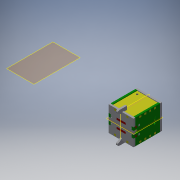
# Autodesk Inventor part: box
Saved by Autodesk Inventor 2019 (Build 230136000, 136)
## iProperties
Created: 2018-09-20
Part Number: box
Material: Générique
Document SubType Name: Modeling
Designer: Jérémy
Density: 1 g/cm^3
Appearance: Par défaut
Author: Jérémy
Autodesk Inventor part; units mm, degrees
(part 1 of 2)
ref_plane "YZ Plane" through (0, 0, 0) normal (1, 0, 0) x (0, 1, 0)
ref_plane "XZ Plane" through (0, 0, 0) normal (0, 1, 0) x (-1, 0, 0)
ref_plane "XY Plane" through (0, 0, 0) normal (0, 0, 1) x (1, 0, 0)
sketch "Esquisse1" plane through (0, 0, 0) normal (0, 0, 1) x (1, 0, 0)
  line L0 (0, 11.8) -> (0, 9.4) projected
  line L1 (0, 11.8) -> (-8.8, 11.8) construction
  line L2 (-8.8, 0) -> (-8.8, 11.8) construction
  line L3 (0, 0) -> (-8.8, 0) projected
  line L4 (0, 2.4) -> (0, 0) projected
  line L5 (0, 2.4) -> (19.5, 2.4) projected
  line L6 (19.5, 9.4) -> (19.5, 2.4) projected
  line L7 (0, 9.4) -> (19.5, 9.4) projected
  line L8 (64, 0) -> (64, 2.4) projected
  line L9 (64, 0) -> (72.8, 0) projected
  line L10 (72.8, 11.8) -> (72.8, 0) construction
  line L11 (64, 11.8) -> (72.8, 11.8) construction
  line L12 (64, 9.4) -> (64, 11.8) projected
  line L13 (64, 9.4) -> (44.5, 9.4) projected
  line L14 (44.5, 2.4) -> (44.5, 9.4) projected
  line L15 (64, 2.4) -> (44.5, 2.4) projected
  line L16 (19.5, 9.4) -> (19.5, 5.9) construction
  line L17 (19.5, 5.9) -> (19.5, 2.4) construction
  line L18 (19.5, 9.4) -> (32, 9.4) construction
  line L19 (32, 9.4) -> (44.5, 9.4) construction
  line L20 (-27.9434, 5.9) -> (85.3545, 5.9) construction
  line L21 (32, 17.9523) -> (32, -8.6548) construction
  line L22 (-8.8, 5.9) -> (-8.8, 11.8)
  line L23 (-2.8, 11.8) -> (-2.8, 21.9)
  line L24 (-2.8, 21.9) -> (17, 21.9)
  line L25 (17, 21.9) -> (17, 15.9)
  line L26 (17, 15.9) -> (32, 15.9)
  line L27 (-2.8, 11.8) -> (-8.8, 11.8)
  circle A0 centre (0.2, 14.8) radius 1.5
  line L28 (64, 11.8) -> (72.8, 11.8) construction
  line L29 (72.8, 0) -> (72.8, 11.8) construction
  line L30 (72.8, 5.9) -> (72.8, 11.8)
  line L31 (66.8, 11.8) -> (66.8, 21.9)
  line L32 (66.8, 21.9) -> (47, 21.9)
  line L33 (47, 21.9) -> (47, 15.9)
  line L34 (47, 15.9) -> (32, 15.9)
  line L35 (66.8, 11.8) -> (72.8, 11.8)
  circle A1 centre (63.8, 14.8) radius 1.5
  line L36 (0, 0) -> (-8.8, 0) construction
  line L37 (64, 0) -> (72.8, 0) construction
  line L38 (-8.8, 5.9) -> (-8.8, 0)
  line L39 (-2.8, 0) -> (-2.8, -10.1)
  line L40 (-2.8, -10.1) -> (17, -10.1)
  line L41 (17, -10.1) -> (17, -4.1)
  line L42 (17, -4.1) -> (32, -4.1)
  line L43 (-2.8, 0) -> (-8.8, 0)
  circle A2 centre (0.2, -3) radius 1.5
  line L44 (64, 0) -> (72.8, 0) construction
  line L45 (66.8, -10.1) -> (47, -10.1)
  line L46 (47, -4.1) -> (32, -4.1)
  line L47 (47, -10.1) -> (47, -4.1)
  circle A3 centre (63.8, -3) radius 1.5
  line L48 (66.8, 0) -> (66.8, -10.1)
  line L49 (66.8, 0) -> (72.8, 0)
  line L50 (72.8, 5.9) -> (72.8, 0)
  point P0 (19.5, 5.9)
  dimension "d0" = 6
  dimension "d1" = 15
  dimension "d2" = 6
  dimension "d3" = 16
  dimension "d4" = 3
  dimension "d5" = 3
  dimension "d6" = 3
  constraints: 70 end point, 17 symmetric about line, 8 point on line, 6 collinear, 4 centre point, 4 perpendicular, 3 midpoint, 2 coincident, 1 horizontal, 1 parallel, 1 vertical, 3 other
  measures "d0" distance of L1.end L23.start
  measures "d1" distance of L25.end L26.end
  measures "d2" distance of L24.end L25.end
  measures "d3" vertical distance of L22.start L23.end
  measures "d4" diameter of A0
  measures "d5" vertical distance of L0.start A0.centre
  measures "d6" horizontal distance of L23.start A0.centre
extrude "Extrusion1" add sketch "Esquisse1" along normal blind 6
ref_plane "Plan de construction1" through (5, 11.8, -9.8) normal (0, 0, -1) x (-1, 0, 0)
sketch "Esquisse2" plane through (5, 11.8, -9.8) normal (0, 0, -1) x (-1, 0, 0)
  circle A0 centre (-58.8, -14.8) radius 1.5 projected
  circle A1 centre (4.8, -14.8) radius 1.5 projected
  circle A2 centre (-58.8, 3) radius 1.5 projected
  circle A3 centre (4.8, 3) radius 1.5 projected
  line L0 (13.8, 0) -> (13.8, -11.8) construction
  line L1 (7.8, 0) -> (13.8, 0) construction
  line L2 (7.8, 10.1) -> (7.8, 0) projected
  line L3 (-12, 10.1) -> (7.8, 10.1) projected
  line L4 (-12, 4.1) -> (-12, 10.1) projected
  line L5 (-42, 4.1) -> (-12, 4.1) projected
  line L6 (-42, 10.1) -> (-42, 4.1) projected
  line L7 (-61.8, 10.1) -> (-42, 10.1) projected
  line L8 (-61.8, 0) -> (-61.8, 10.1) construction
  line L9 (-67.8, 0) -> (-61.8, 0) construction
  line L10 (-67.8, -11.8) -> (-67.8, 0) projected
  line L11 (-61.8, -11.8) -> (-67.8, -11.8) construction
  line L12 (-61.8, -21.9) -> (-61.8, -11.8) construction
  line L13 (-42, -21.9) -> (-61.8, -21.9) projected
  line L14 (-42, -15.9) -> (-42, -21.9) projected
  line L15 (-12, -15.9) -> (-42, -15.9) construction
  line L16 (-12, -21.9) -> (-12, -15.9) projected
  line L17 (7.8, -21.9) -> (-12, -21.9) projected
  line L18 (7.8, -11.8) -> (7.8, -21.9) construction
  line L19 (13.8, -11.8) -> (7.8, -11.8) construction
  line L20 (-67.8, -11.8) -> (-67.8, 0) construction
  line L21 (-67.8, -11.8) -> (-67.8, -5.9) construction
  line L22 (-67.8, -5.9) -> (-67.8, 0) construction
  line L23 (23.1291, -5.9) -> (-93.9049, -5.9) construction
  line L24 (-12, -15.9) -> (-42, -15.9) construction
  line L25 (-12, -15.9) -> (-27, -15.9) construction
  line L26 (-27, -15.9) -> (-42, -15.9) construction
  line L27 (-27, -48.0449) -> (-27, 22.4449) construction
  line L28 (13.8, -21.4) -> (13.8, -16.4)
  line L29 (7.8, -21.9) -> (-12, -21.9) projected
  line L30 (13.3, -21.9) -> (-12, -21.9)
  line L31 (-12, -21.9) -> (-12, -15.9)
  line L32 (-27, -15.9) -> (-12, -15.9)
  line L33 (-12, -15.9) -> (18.1212, -15.9) construction
  line L34 (-9.5, -11.8) -> (-9.5, 0) construction
  line L35 (-9.5, 0) -> (-14.5, 0) construction
  line L36 (-14.5, -11.8) -> (-14.5, 0) construction
  line L37 (-9.5, -11.8) -> (-14.5, -11.8) construction
  line L38 (-44.5, 0) -> (-44.5, -11.8) construction
  line L39 (-44.5, -11.8) -> (-39.5, -11.8) construction
  line L40 (-39.5, 0) -> (-39.5, -11.8) construction
  line L41 (-44.5, 0) -> (-39.5, 0) construction
  line L42 (-27, -12.8) -> (-7.5, -12.8)
  line L43 (-7.5, -12.8) -> (-7.5, -12.8)
  line L44 (-7.5, -12.8) -> (-7.5, -5.9)
  circle A4 centre (-58.8, -14.8) radius 1.5
  line L45 (-42, -15.9) -> (-12, -15.9) construction
  line L46 (-42, -21.9) -> (-42, -15.9)
  line L47 (-61.8, -21.9) -> (-42, -21.9)
  line L48 (-42, -15.9) -> (-12, -15.9) construction
  line L49 (-42, -15.9) -> (-27, -15.9) construction
  line L50 (-67.3, -21.9) -> (-42, -21.9)
  line L51 (-27, -15.9) -> (-42, -15.9)
  line L52 (-27, -12.8) -> (-46.5, -12.8)
  line L53 (-46.5, -12.8) -> (-46.5, -5.9)
  circle A5 centre (-58.8, 3) radius 1.5
  circle A6 centre (4.8, 3) radius 1.5
  line L54 (-42.5, 10.1) -> (-61.8, 10.1)
  line L55 (-42, 4.1) -> (-42, 9.6)
  line L56 (-12, 9.6) -> (-12, 4.1)
  line L57 (7.8, 10.1) -> (-11.5, 10.1)
  line L58 (7.8, 0) -> (7.8, 10.1) construction
  line L59 (-12, 4.1) -> (-27, 4.1) construction
  line L60 (7.8, 10.1) -> (-12, 10.1)
  line L61 (13.3, 10.1) -> (-12, 10.1)
  line L62 (-12, 10.1) -> (-12, 4.1)
  line L63 (-27, 4.1) -> (-12, 4.1)
  line L64 (-27, 1) -> (-7.5, 1)
  line L65 (-7.5, 1) -> (-7.5, -5.9)
  line L66 (-27, 4.1) -> (-42, 4.1)
  line L67 (-67.3, 10.1) -> (-42, 10.1)
  line L68 (-46.5, 1) -> (-46.5, -5.9)
  line L69 (-27, 1) -> (-46.5, 1)
  circle A7 centre (-58.8, 3) radius 1.5
  line L70 (7.8, -5.9) -> (7.8, -15.9)
  line L71 (7.8, -11.8) -> (7.8, -21.9) construction
  line L72 (13.3, -15.9) -> (7.8, -15.9)
  line L73 (-67.8, -21.4) -> (-67.8, -16.4)
  line L74 (-61.8, -5.9) -> (-61.8, -15.9)
  line L75 (-67.3, -15.9) -> (-61.8, -15.9)
  line L76 (13.8, 9.6) -> (13.8, 4.6)
  line L77 (7.8, -5.9) -> (7.8, 4.1)
  line L78 (13.3, 4.1) -> (7.8, 4.1)
  line L79 (-67.8, 9.6) -> (-67.8, 4.6)
  line L80 (-67.3, 4.1) -> (-61.8, 4.1)
  line L81 (-61.8, -5.9) -> (-61.8, 4.1)
  line L82 (-67.3, -21.9) -> (-67.8, -21.4)
  line L83 (-67.8, -16.4) -> (-67.3, -15.9)
  line L84 (-67.3, 4.1) -> (-67.8, 4.6)
  line L85 (-67.8, 9.6) -> (-67.3, 10.1)
  line L86 (-42.5, 10.1) -> (-42, 9.6)
  line L87 (-12, 9.6) -> (-11.5, 10.1)
  line L88 (13.3, 10.1) -> (13.8, 9.6)
  line L89 (13.3, 4.1) -> (13.8, 4.6)
  line L90 (13.3, -15.9) -> (13.8, -16.4)
  line L91 (13.3, -21.9) -> (13.8, -21.4)
  point P0 (5, -11.8)
  point P1 (13.8, -21.9)
  point P2 (13.8, -15.9)
  point P3 (7.8, -16.85)
  point P4 (-67.8, -21.9)
  point P5 (13.8, 10.1)
  point P6 (-67.8, 10.1)
  point P7 (-67.8, -15.9)
  point P8 (13.8, 4.1)
  point P9 (-67.8, 4.1)
  dimension "d9" = 2
  dimension "d10" = 1
  dimension "d83" = 0.5
  dimension "d84" = 0.5
  dimension "d85" = 0.5
  dimension "d86" = 0.5
  dimension "d87" = 0.5
  dimension "d88" = 0.5
  dimension "d89" = 0.5
  dimension "d90" = 0.5
  dimension "d91" = 0.5
  dimension "d92" = 0.5
  dimension "d93" = 0.5
  dimension "d94" = 0.5
  dimension "d95" = 0.5
  dimension "d96" = 0.5
  dimension "d97" = 0.5
  dimension "d98" = 0.5
  dimension "d99" = 0.5
  dimension "d100" = 0.5
  dimension "d101" = 0.5
  dimension "d102" = 0.5
  constraints: 120 end point, 29 point on line, 26 symmetric about line, 7 collinear, 4 centre point, 4 midpoint, 3 perpendicular, 2 coincident, 2 parallel, 1 horizontal, 1 vertical, 4 other
  measures "d9" distance between parallel lines of L44 L34
  measures "d10" distance between parallel lines of L37 L42
  measures "d83" distance of L50.start point (-67.8, -21.9)
  measures "d84" distance of L73.start point (-67.8, -21.9)
  measures "d85" distance of L73.end point (-67.8, -15.9)
  measures "d86" distance of L75.start point (-67.8, -15.9)
  measures "d87" distance of L80.start point (-67.8, 4.1)
  measures "d88" distance of L79.end point (-67.8, 4.1)
  measures "d89" distance of L79.start point (-67.8, 10.1)
  measures "d90" distance of L67.start point (-67.8, 10.1)
  measures "d91" distance of L54.start L6.start
  measures "d92" distance of L55.end L6.start
  measures "d93" distance of L56.start L3.start
  measures "d94" distance of L57.end L3.start
  measures "d95" distance of L61.start point (13.8, 10.1)
  measures "d96" distance of L76.start point (13.8, 10.1)
  measures "d97" distance of L78.start point (13.8, 4.1)
  measures "d98" distance of L76.end point (13.8, 4.1)
  measures "d99" distance of L72.start point (13.8, -15.9)
  measures "d100" distance of L28.end point (13.8, -15.9)
  measures "d101" distance of L30.start point (13.8, -21.9)
  measures "d102" distance of L28.start point (13.8, -21.9)
extrude "Extrusion2" add sketch "Esquisse2" along normal blind 6
ref_plane "Plan de construction2" through (17, 5.9, -9.8) normal (0, 1, 0) x (1, 0, 0)
sketch "Esquisse6" plane through (-10.8, 21.9, -9.8) normal (0, 1, 0) x (1, 0, 0)
  line L0 (27.8, 0) -> (57.8, 0) construction
  line L1 (57.8, 0) -> (57.8, 6) construction
  line L2 (27.8, 6) -> (57.8, 6) construction
  line L3 (27.8, 0) -> (27.8, 6) construction
  line L4 (27.8, 0) -> (27.8, 6) construction
  line L5 (57.8, 0) -> (83.1, 0) construction
  line L6 (57.8, 6) -> (83.1, 6) construction
  line L7 (57.8, 0) -> (57.8, 6) construction
  line L8 (77.6, -9.8) -> (57.8, -9.8) construction
  line L9 (57.8, -9.8) -> (57.8, -15.8) construction
  line L10 (77.6, -15.8) -> (57.8, -15.8) construction
  line L11 (77.6, -9.8) -> (77.6, -15.8) construction
  line L12 (57.8, -9.8) -> (27.8, -9.8) construction
  line L13 (27.8, -9.8) -> (27.8, -15.8) construction
  line L14 (57.8, -15.8) -> (27.8, -15.8) construction
  line L15 (57.8, -9.8) -> (57.8, -15.8) construction
  line L16 (27.8, -9.8) -> (8, -9.8) construction
  line L17 (8, -9.8) -> (8, -15.8) construction
  line L18 (27.8, -15.8) -> (8, -15.8) construction
  line L19 (27.8, -9.8) -> (27.8, -15.8) construction
  line L20 (27.8, -9.8) -> (8, -9.8) projected
  line L21 (8, -9.8) -> (2, -9.8)
  line L22 (8, -9.8) -> (2, -9.8) projected
  line L23 (2, -9.8) -> (2, -6)
  line L24 (27.8, 0) -> (27.8, 6) projected
  line L25 (27.8, 0) -> (27.8, 6)
  line L26 (57.8, 0) -> (57.8, 6) projected
  line L27 (57.8, 6) -> (57.8, 0)
  line L28 (8, -9.8) -> (27.8, -9.8)
  line L29 (27.8, -9.8) -> (27.8, -15.8)
  line L30 (27.8, -15.8) -> (8, -15.8) construction
  line L31 (57.8, -15.8) -> (57.8, -9.8)
  line L32 (57.8, -9.8) -> (57.8, -15.8) projected
  line L33 (57.8, -9.8) -> (83.6, -9.8)
  line L34 (83.6, -9.8) -> (83.6, -6)
  line L35 (83.6, -6) -> (77.6, -6)
  line L36 (77.6, -6) -> (77.6, 0)
  line L37 (57.8, 0) -> (83.1, 0) construction
  line L38 (57.8, 0) -> (77.6, 0)
  line L39 (27.8, 0) -> (27.8, 6) projected
  line L40 (27.8, 6) -> (42.8, 6) construction
  line L41 (42.8, 6) -> (57.8, 6) construction
  line L42 (42.8, 17.4784) -> (42.8, -29.8094) construction
  line L43 (50.3, 16.5) -> (50.3, 6)
  line L44 (57.8, 6) -> (50.3, 6)
  line L45 (35.8, 17) -> (42.8, 17)
  line L46 (42.8, 17) -> (49.8, 17)
  line L47 (27.8, 6) -> (57.8, 6) projected
  line L48 (27.8, 6) -> (35.3, 6)
  line L49 (35.3, 16.5) -> (35.3, 6)
  line L50 (57.8, -15.8) -> (77.6, -15.8) construction
  line L51 (27.8, -15.8) -> (57.8, -15.8)
  line L52 (8, -9.8) -> (8, -15.8) projected
  line L53 (57.8, 0) -> (27.8, 0) projected
  line L54 (27.8, 0) -> (2.5, 0) construction
  line L55 (2, -6) -> (8, -6)
  line L56 (8, -6) -> (8, 0)
  line L57 (8, 0) -> (27.8, 0)
  line L58 (83.1, 0) -> (83.1, 6) projected
  line L59 (2, 0) -> (2, 6) projected
  line L60 (83.6, 0) -> (83.6, 6) projected
  line L61 (35.8, 17) -> (35.3, 16.5)
  line L62 (49.8, 17) -> (50.3, 16.5)
  point P0 (10.8, -9.8)
  point P1 (83.6, 0)
  point P2 (35.3, 17)
  point P3 (50.3, 17)
  dimension "d28" = 6
  dimension "d29" = 6
  dimension "d33" = 11
  dimension "d35" = 7.5
  dimension "d103" = 0.5
  dimension "d104" = 0.5
  dimension "d105" = 0.5
  dimension "d106" = 0.5
  constraints: 60 end point, 9 perpendicular, 7 collinear, 7 point on line, 5 horizontal, 5 parallel, 4 equal length, 2 midpoint, 1 coincident, 2 other
  measures "d28" distance of L35.end L36.end
  measures "d29" distance of L34.end L35.end
  measures "d33" distance of point (50.3, 17) L43.end
  measures "d35" distance of L45.end point (50.3, 17)
  measures "d103" distance of L45.start point (35.3, 17)
  measures "d104" distance of L49.start point (35.3, 17)
  measures "d105" distance of L46.end point (50.3, 17)
  measures "d106" distance of L43.start point (50.3, 17)
extrude "Extrusion4" add sketch "Esquisse6" against normal blind 6 separate body
mirror "Symétrie2" about plane through (17, 5.9, -9.8) normal (0, 1, 0) of "Extrusion4" bodies 2
sketch "Esquisse7" plane through (0, 0, 6) normal (0, 0, 1) x (1, 0, 0)
  circle A0 centre (63.8, -3) radius 1.5 construction
  circle A1 centre (0.2, -3) radius 1.5 construction
  circle A2 centre (63.8, 14.8) radius 1.5 construction
  circle A3 centre (0.2, 14.8) radius 1.5 construction
  line L0 (-8.8, 11.8) -> (-8.8, 0) construction
  line L1 (-8.8, 0) -> (-2.8, 0) construction
  line L2 (-2.8, 0) -> (-2.8, -10.1) construction
  line L3 (-2.8, -10.1) -> (17, -10.1) construction
  line L4 (17, -10.1) -> (17, -4.1) construction
  line L5 (17, -4.1) -> (47, -4.1) construction
  line L6 (47, -4.1) -> (47, -10.1) construction
  line L7 (47, -10.1) -> (66.8, -10.1) construction
  line L8 (66.8, -10.1) -> (66.8, 0) construction
  line L9 (66.8, 0) -> (72.8, 0) construction
  line L10 (72.8, 0) -> (72.8, 11.8) construction
  line L11 (72.8, 11.8) -> (66.8, 11.8) construction
  line L12 (66.8, 11.8) -> (66.8, 21.9) construction
  line L13 (66.8, 21.9) -> (47, 21.9) construction
  line L14 (47, 21.9) -> (47, 15.9) construction
  line L15 (47, 15.9) -> (17, 15.9) construction
  line L16 (17, 15.9) -> (17, 21.9) construction
  line L17 (17, 21.9) -> (-2.8, 21.9) construction
  line L18 (-2.8, 21.9) -> (-2.8, 11.8) construction
  line L19 (-2.8, 11.8) -> (-8.8, 11.8) construction
  line L20 (-2.8, 21.9) -> (-8.8, 21.9)
  line L21 (-8.8, 21.9) -> (-8.8, 46.7)
  line L22 (-8.8, 46.7) -> (72.8, 46.7)
  line L23 (72.8, 46.7) -> (72.8, 21.9)
  line L24 (72.8, 21.9) -> (66.8, 21.9)
  line L25 (17, 21.9) -> (-2.8, 21.9) construction
  line L26 (66.8, 11.8) -> (66.8, 21.9) construction
  line L27 (-8.8, 11.8) -> (-8.8, 0) construction
  line L28 (66.8, 21.9) -> (47, 21.9) construction
  line L29 (-25.12, 5.9) -> (89.12, 5.9) projected
  line L30 (8.1, 44.7) -> (15.1, 44.7)
  line L31 (15.1, 44.7) -> (15.1, 38.7)
  line L32 (15.1, 38.7) -> (8.1, 38.7)
  line L33 (8.1, 38.7) -> (8.1, 44.7)
  line L34 (48.9, 44.7) -> (55.9, 44.7)
  line L35 (55.9, 44.7) -> (55.9, 38.7)
  line L36 (55.9, 38.7) -> (48.9, 38.7)
  line L37 (48.9, 38.7) -> (48.9, 44.7)
  line L38 (17, 21.9) -> (-2.8, 21.9) projected
  line L39 (-2.8, 21.9) -> (66.8, 21.9)
  line L40 (-2.8, -10.1) -> (-8.8, -10.1)
  line L41 (-8.8, -10.1) -> (-8.8, -34.9)
  line L42 (-8.8, -34.9) -> (72.8, -34.9)
  line L43 (72.8, -34.9) -> (72.8, -10.1)
  line L44 (72.8, -10.1) -> (66.8, -10.1)
  line L45 (8.1, -32.9) -> (15.1, -32.9)
  line L46 (15.1, -32.9) -> (15.1, -26.9)
  line L47 (15.1, -26.9) -> (8.1, -26.9)
  line L48 (8.1, -26.9) -> (8.1, -32.9)
  line L49 (48.9, -32.9) -> (55.9, -32.9)
  line L50 (55.9, -32.9) -> (55.9, -26.9)
  line L51 (55.9, -26.9) -> (48.9, -26.9)
  line L52 (48.9, -26.9) -> (48.9, -32.9)
  line L53 (-2.8, -10.1) -> (66.8, -10.1)
  line L54 (49.6, 38.7) -> (49.6, 38.9)
  line L55 (49.6, 38.9) -> (50.6, 38.9)
  line L56 (50.6, 38.9) -> (50.6, 38.7)
  line L57 (54.2, 38.7) -> (54.2, 38.9)
  line L58 (54.2, 38.9) -> (55.2, 38.9)
  line L59 (55.2, 38.9) -> (55.2, 38.7)
  line L60 (51.9, 44.7) -> (51.9, 44.5)
  line L61 (51.9, 44.5) -> (52.9, 44.5)
  line L62 (52.9, 44.5) -> (52.9, 44.7)
  line L63 (8.8, 38.7) -> (8.8, 38.9)
  line L64 (8.8, 38.9) -> (9.8, 38.9)
  line L65 (9.8, 38.9) -> (9.8, 38.7)
  line L66 (13.4, 38.7) -> (13.4, 38.9)
  line L67 (13.4, 38.9) -> (14.4, 38.9)
  line L68 (14.4, 38.9) -> (14.4, 38.7)
  line L69 (11.1, 44.7) -> (11.1, 44.5)
  line L70 (11.1, 44.5) -> (12.1, 44.5)
  line L71 (12.1, 44.5) -> (12.1, 44.7)
  line L72 (49.6, -32.9) -> (49.6, -32.7)
  line L73 (49.6, -32.7) -> (50.6, -32.7)
  line L74 (50.6, -32.7) -> (50.6, -32.9)
  line L75 (54.2, -32.9) -> (54.2, -32.7)
  line L76 (54.2, -32.7) -> (55.2, -32.7)
  line L77 (55.2, -32.7) -> (55.2, -32.9)
  line L78 (51.9, -26.9) -> (51.9, -27.1)
  line L79 (51.9, -27.1) -> (52.9, -27.1)
  line L80 (52.9, -27.1) -> (52.9, -26.9)
  line L81 (8.8, -32.9) -> (8.8, -32.7)
  line L82 (8.8, -32.7) -> (9.8, -32.7)
  line L83 (9.8, -32.7) -> (9.8, -32.9)
  line L84 (13.4, -32.9) -> (13.4, -32.7)
  line L85 (13.4, -32.7) -> (14.4, -32.7)
  line L86 (14.4, -32.7) -> (14.4, -32.9)
  line L87 (11.1, -26.9) -> (11.1, -27.1)
  line L88 (11.1, -27.1) -> (12.1, -27.1)
  line L89 (12.1, -27.1) -> (12.1, -26.9)
  point P0 (0, 0)
  dimension "d36" = 6
  dimension "d37" = 6
  dimension "d38" = 40.8
  dimension "d39" = 16.9
  dimension "d40" = 16.9
  dimension "d41" = 7
  dimension "d43" = 7
  dimension "d45" = 2
  dimension "d46" = 6
  dimension "d107" = 0.2
  dimension "d108" = 1
  dimension "d109" = 0.7
  dimension "d110" = 0.7
  dimension "d111" = 1
  dimension "d112" = 3
  dimension "d113" = 1
  dimension "d114" = 0.2
  dimension "d115" = 1
  dimension "d116" = 0.2
  dimension "d117" = 0.2
  dimension "d118" = 1
  dimension "d119" = 0.2
  dimension "d120" = 3
  dimension "d121" = 0.7
  dimension "d122" = 1
  dimension "d123" = 0.7
  dimension "d124" = 1
  dimension "d125" = 1
  dimension "d126" = 1
  dimension "d127" = 0.2
  dimension "d128" = 0.2
  dimension "d129" = 0.7
  dimension "d130" = 0.7
  dimension "d131" = 3
  dimension "d132" = 1
  dimension "d133" = 1
  dimension "d134" = 1
  dimension "d135" = 0.2
  dimension "d136" = 0.2
  dimension "d137" = 3
  dimension "d138" = 0.7
  dimension "d139" = 0.7
  constraints: 128 end point, 31 perpendicular, 30 point on line, 12 symmetric about line, 9 parallel, 7 collinear, 2 horizontal
  measures "d36" distance of L23.end L12.end
  measures "d37" distance of L17.end L20.end
  measures "d38" distance from line of L29 L21.end
  measures "d39" horizontal distance of L30.start L21.end
  measures "d40" horizontal distance of L22.end L34.end
  measures "d41" distance of L34.start L34.end
  measures "d43" distance of L30.start L30.end
  measures "d45" vertical distance of L34.end L22.end
  measures "d46" distance of L34.end L35.end
  measures "d107" distance of L55.end L56.end
  measures "d108" distance of L54.end L55.end
  measures "d109" distance from line of L37 L54.end
  measures "d110" horizontal distance of L35.end L58.end
  measures "d111" distance of L57.end L58.end
  measures "d112" horizontal distance of L34.start L60.end
  measures "d113" distance of L60.end L61.end
  measures "d114" distance of L61.end L62.end
  measures "d115" distance of L66.end L67.end
  measures "d116" distance of L67.end L68.end
  measures "d117" distance of L64.end L65.end
  measures "d118" distance of L69.end L70.end
  measures "d119" distance of L70.end L71.end
  measures "d120" horizontal distance of L30.start L69.end
  measures "d121" horizontal distance of L32.end L63.end
  measures "d122" distance of L63.end L64.end
  measures "d123" horizontal distance of L31.end L67.end
  measures "d124" distance of L72.end L73.end
  measures "d125" distance of L75.end L76.end
  measures "d126" distance of L78.end L79.end
  measures "d127" distance of L78.start L78.end
  measures "d128" distance of L72.start L72.end
  measures "d129" horizontal distance of L52.end L72.end
  measures "d130" horizontal distance of L49.end L76.end
  measures "d131" horizontal distance of L52.start L78.end
  measures "d132" distance of L81.end L82.end
  measures "d133" distance of L84.end L85.end
  measures "d134" distance of L87.end L88.end
  measures "d135" distance of L82.end L83.end
  measures "d136" distance of L88.end L89.end
  measures "d137" horizontal distance of L48.start L87.end
  measures "d138" horizontal distance of L45.start L81.end
  measures "d139" horizontal distance of L46.start L85.end
extrude "Extrusion5" add sketch "Esquisse7" against normal blind 6 contours L20 L21 L22 L23 L24 L39 L38 | L30 L71 L70 L69 | L63 L64 L65 L32 | L66 L67 L68 L32 | L34 L62 L61 L60 | L54 L55 L56 L36 | L57 L58 L59 L36 | L53 L44 L43 L42 L41 L40 | L81 L82 L83 L45 | L47 L89 L88 L87 | L84 L85 L86 L45 | L72 L73 L74 L49 | L51 L80 L79 L78 | L75 L76 L77 L49 bodies 1
sketch "Esquisse8" plane through (72.8, -14.05, -9.8) normal (1, 0, 0) x (0, 0, -1)
  line L0 (-15.8, 35.95) -> (-15.8, 60.75) construction
  line L1 (-15.8, 35.95) -> (-9.8, 35.95) construction
  line L2 (-9.8, 60.75) -> (-9.8, 35.95) construction
  line L3 (-15.8, 60.75) -> (-9.8, 60.75) construction
  line L4 (-9.8, 60.75) -> (-9.8, 35.95) projected
  line L5 (-9.8, 35.95) -> (-9.8, 60.75)
  line L6 (-9.8, 60.75) -> (71.8, 60.75)
  line L7 (71.8, 60.75) -> (71.8, -20.85)
  line L8 (-6, 35.95) -> (-6, 29.95) projected
  line L9 (-9.8, 35.95) -> (-6, 35.95)
  line L10 (-6, 35.95) -> (-6, 29.95)
  line L11 (-5.9724, 20.85) -> (-3.8276, 20.85) construction
  arc A0 (-5.9724, 20.85) -> (-3.8276, 20.85) centre (-4.9, 19.95) ccw construction
  line L12 (-9.8, 14.05) -> (0, 14.05) projected
  line L13 (0, 14.05) -> (0, 25.85) construction
  line L14 (0, 25.85) -> (-9.8, 25.85) projected
  line L15 (-9.8, 25.85) -> (-9.8, 14.05) construction
  line L16 (-9.8, 29.95) -> (-9.8, 35.95)
  line L17 (-9.8, 35.95) -> (-9.8, 60.75) projected
  line L18 (-9.8, 35.95) -> (-15.8, 35.95) projected
  line L19 (-9.8, 35.95) -> (-15.8, 35.95)
  line L20 (-6, 29.95) -> (-9.8, 29.95)
  line L21 (-15.8, 25.85) -> (-15.8, 35.95) projected
  line L22 (-15.8, 35.95) -> (-15.8, 25.85)
  line L23 (-15.8, 25.85) -> (0, 25.85)
  line L24 (0, 25.85) -> (0, 14.05)
  line L25 (-9.8, 14.05) -> (-15.8, 14.05) projected
  line L26 (0, 14.05) -> (-15.8, 14.05)
  line L27 (-15.8, 3.95) -> (-9.8, 3.95) projected
  line L28 (-15.8, 14.05) -> (-15.8, 3.95)
  line L29 (-15.8, 3.95) -> (-9.8, 3.95)
  line L30 (-9.8, 3.95) -> (-9.8, 9.95)
  line L31 (-9.8, 9.95) -> (-6, 9.95)
  line L32 (-6, 9.95) -> (-6, 3.95)
  line L33 (-6, 3.95) -> (-9.8, 3.95)
  line L34 (-9.8, 3.95) -> (-9.8, -20.85) projected
  line L35 (-9.8, 3.95) -> (-9.8, -20.85)
  line L36 (-9.8, -20.85) -> (71.8, -20.85)
  line L37 (51.98, 58.75) -> (51.98, 52.75)
  line L38 (58.98, 52.75) -> (58.98, 58.75)
  line L39 (35.66, 58.75) -> (35.66, 52.75)
  line L40 (42.66, 52.75) -> (42.66, 58.75)
  line L41 (19.34, 58.75) -> (19.34, 52.75)
  line L42 (26.34, 52.75) -> (26.34, 58.75)
  line L43 (3.02, 58.75) -> (3.02, 52.75)
  line L44 (10.02, 52.75) -> (10.02, 58.75)
  line L45 (71.8, 60.75) -> (71.8, 19.95) construction
  line L46 (71.8, 19.95) -> (71.8, -20.85) construction
  line L47 (99.7668, 19.95) -> (-38.6009, 19.95) construction
  line L48 (-6, 3.95) -> (-6, 9.95) projected
  line L49 (0, 29.95) -> (6, 29.95) projected
  line L50 (6, 29.95) -> (0, 29.95)
  line L51 (0, 35.95) -> (0, 29.95) construction
  line L52 (0, 35.95) -> (6, 35.95) projected
  line L53 (0, 35.95) -> (6, 35.95)
  line L54 (0, 4.45) -> (0, 3.95) projected
  line L55 (6, 3.95) -> (0, 3.95)
  line L56 (0, 9.95) -> (6, 9.95)
  line L57 (6, 3.95) -> (6, 9.95) construction
  line L58 (0, 3.95) -> (6, 3.95) projected
  line L59 (6, 29.95) -> (6, 35.95) construction
  line L60 (6, 35.25) -> (5.8, 35.25)
  line L61 (5.8, 35.25) -> (5.8, 34.25)
  line L62 (5.8, 34.25) -> (6, 34.25)
  line L63 (6, 31.65) -> (5.8, 31.65)
  line L64 (5.8, 31.65) -> (5.8, 30.65)
  line L65 (5.8, 30.65) -> (6, 30.65)
  line L66 (0, 33.45) -> (0.2, 33.45)
  line L67 (0.2, 33.45) -> (0.2, 32.45)
  line L68 (0.2, 32.45) -> (0, 32.45)
  line L69 (0, 29.95) -> (0, 35.95) projected
  line L70 (6, 9.95) -> (6, 3.95) construction
  line L71 (6, 9.25) -> (5.8, 9.25)
  line L72 (5.8, 9.25) -> (5.8, 8.25)
  line L73 (5.8, 8.25) -> (6, 8.25)
  line L74 (6, 5.65) -> (5.8, 5.65)
  line L75 (5.8, 5.65) -> (5.8, 4.65)
  line L76 (5.8, 4.65) -> (6, 4.65)
  line L77 (0, 7.45) -> (0.2, 7.45)
  line L78 (0.2, 7.45) -> (0.2, 6.45)
  line L79 (0.2, 6.45) -> (0, 6.45)
  line L80 (0, 9.95) -> (0, 3.95) construction
  line L81 (58.28, 58.75) -> (58.28, 58.55)
  line L82 (58.28, 58.55) -> (57.28, 58.55)
  line L83 (57.28, 58.55) -> (57.28, 58.75)
  line L84 (53.68, 58.75) -> (53.68, 58.55)
  line L85 (53.68, 58.55) -> (52.68, 58.55)
  line L86 (52.68, 58.55) -> (52.68, 58.75)
  line L87 (55.98, 52.75) -> (55.98, 52.95)
  line L88 (55.98, 52.95) -> (54.98, 52.95)
  line L89 (54.98, 52.95) -> (54.98, 52.75)
  line L90 (41.96, 58.75) -> (41.96, 58.55)
  line L91 (41.96, 58.55) -> (40.96, 58.55)
  line L92 (40.96, 58.55) -> (40.96, 58.75)
  line L93 (37.36, 58.75) -> (37.36, 58.55)
  line L94 (37.36, 58.55) -> (36.36, 58.55)
  line L95 (36.36, 58.55) -> (36.36, 58.75)
  line L96 (39.66, 52.75) -> (39.66, 52.95)
  line L97 (39.66, 52.95) -> (38.66, 52.95)
  line L98 (38.66, 52.95) -> (38.66, 52.75)
  line L99 (25.64, 58.75) -> (25.64, 58.55)
  line L100 (25.64, 58.55) -> (24.64, 58.55)
  line L101 (24.64, 58.55) -> (24.64, 58.75)
  line L102 (21.04, 58.75) -> (21.04, 58.55)
  line L103 (21.04, 58.55) -> (20.04, 58.55)
  line L104 (20.04, 58.55) -> (20.04, 58.75)
  line L105 (22.34, 52.75) -> (22.34, 52.95)
  line L106 (22.34, 52.95) -> (23.34, 52.95)
  line L107 (23.34, 52.95) -> (23.34, 52.75)
  line L108 (9.32, 58.75) -> (9.32, 58.55)
  line L109 (9.32, 58.55) -> (8.32, 58.55)
  line L110 (8.32, 58.55) -> (8.32, 58.75)
  line L111 (4.72, 58.75) -> (4.72, 58.55)
  line L112 (4.72, 58.55) -> (3.72, 58.55)
  line L113 (3.72, 58.55) -> (3.72, 58.75)
  line L114 (7.02, 52.75) -> (7.02, 52.95)
  line L115 (7.02, 52.95) -> (6.02, 52.95)
  line L116 (6.02, 52.95) -> (6.02, 52.75)
  line L117 (58.98, 58.75) -> (58.28, 58.75)
  line L118 (51.98, 52.75) -> (54.98, 52.75)
  line L119 (55.98, 52.75) -> (58.98, 52.75)
  line L120 (57.28, 58.75) -> (53.68, 58.75)
  line L121 (52.68, 58.75) -> (51.98, 58.75)
  line L122 (42.66, 58.75) -> (41.96, 58.75)
  line L123 (35.66, 52.75) -> (38.66, 52.75)
  line L124 (39.66, 52.75) -> (42.66, 52.75)
  line L125 (40.96, 58.75) -> (37.36, 58.75)
  line L126 (36.36, 58.75) -> (35.66, 58.75)
  line L127 (26.34, 58.75) -> (25.64, 58.75)
  line L128 (19.34, 52.75) -> (22.34, 52.75)
  line L129 (23.34, 52.75) -> (26.34, 52.75)
  line L130 (24.64, 58.75) -> (21.04, 58.75)
  line L131 (20.04, 58.75) -> (19.34, 58.75)
  line L132 (3.02, 52.75) -> (6.02, 52.75)
  line L133 (7.02, 52.75) -> (10.02, 52.75)
  line L134 (10.02, 58.75) -> (9.32, 58.75)
  line L135 (8.32, 58.75) -> (4.72, 58.75)
  line L136 (3.72, 58.75) -> (3.02, 58.75)
  line L137 (51.98, -18.85) -> (51.98, -12.85)
  line L138 (58.98, -12.85) -> (58.98, -18.85)
  line L139 (35.66, -18.85) -> (35.66, -12.85)
  line L140 (42.66, -12.85) -> (42.66, -18.85)
  line L141 (19.34, -18.85) -> (19.34, -12.85)
  line L142 (26.34, -12.85) -> (26.34, -18.85)
  line L143 (3.02, -18.85) -> (3.02, -12.85)
  line L144 (10.02, -12.85) -> (10.02, -18.85)
  line L145 (58.28, -18.85) -> (58.28, -18.65)
  line L146 (58.28, -18.65) -> (57.28, -18.65)
  line L147 (57.28, -18.65) -> (57.28, -18.85)
  line L148 (53.68, -18.85) -> (53.68, -18.65)
  line L149 (53.68, -18.65) -> (52.68, -18.65)
  line L150 (52.68, -18.65) -> (52.68, -18.85)
  line L151 (55.98, -12.85) -> (55.98, -13.05)
  line L152 (55.98, -13.05) -> (54.98, -13.05)
  line L153 (54.98, -13.05) -> (54.98, -12.85)
  line L154 (41.96, -18.85) -> (41.96, -18.65)
  line L155 (41.96, -18.65) -> (40.96, -18.65)
  line L156 (40.96, -18.65) -> (40.96, -18.85)
  line L157 (37.36, -18.85) -> (37.36, -18.65)
  line L158 (37.36, -18.65) -> (36.36, -18.65)
  line L159 (36.36, -18.65) -> (36.36, -18.85)
  line L160 (39.66, -12.85) -> (39.66, -13.05)
  line L161 (39.66, -13.05) -> (38.66, -13.05)
  line L162 (38.66, -13.05) -> (38.66, -12.85)
  line L163 (25.64, -18.85) -> (25.64, -18.65)
  line L164 (25.64, -18.65) -> (24.64, -18.65)
  line L165 (24.64, -18.65) -> (24.64, -18.85)
  line L166 (21.04, -18.85) -> (21.04, -18.65)
  line L167 (21.04, -18.65) -> (20.04, -18.65)
  line L168 (20.04, -18.65) -> (20.04, -18.85)
  line L169 (22.34, -12.85) -> (22.34, -13.05)
  line L170 (22.34, -13.05) -> (23.34, -13.05)
  line L171 (23.34, -13.05) -> (23.34, -12.85)
  line L172 (9.32, -18.85) -> (9.32, -18.65)
  line L173 (9.32, -18.65) -> (8.32, -18.65)
  line L174 (8.32, -18.65) -> (8.32, -18.85)
  line L175 (4.72, -18.85) -> (4.72, -18.65)
  line L176 (4.72, -18.65) -> (3.72, -18.65)
  line L177 (3.72, -18.65) -> (3.72, -18.85)
  line L178 (7.02, -12.85) -> (7.02, -13.05)
  line L179 (7.02, -13.05) -> (6.02, -13.05)
  line L180 (6.02, -13.05) -> (6.02, -12.85)
  line L181 (58.98, -18.85) -> (58.28, -18.85)
  line L182 (51.98, -12.85) -> (54.98, -12.85)
  line L183 (55.98, -12.85) -> (58.98, -12.85)
  line L184 (57.28, -18.85) -> (53.68, -18.85)
  line L185 (52.68, -18.85) -> (51.98, -18.85)
  line L186 (42.66, -18.85) -> (41.96, -18.85)
  line L187 (35.66, -12.85) -> (38.66, -12.85)
  line L188 (39.66, -12.85) -> (42.66, -12.85)
  line L189 (40.96, -18.85) -> (37.36, -18.85)
  line L190 (36.36, -18.85) -> (35.66, -18.85)
  line L191 (26.34, -18.85) -> (25.64, -18.85)
  line L192 (19.34, -12.85) -> (22.34, -12.85)
  line L193 (23.34, -12.85) -> (26.34, -12.85)
  line L194 (24.64, -18.85) -> (21.04, -18.85)
  line L195 (20.04, -18.85) -> (19.34, -18.85)
  line L196 (3.02, -12.85) -> (6.02, -12.85)
  line L197 (7.02, -12.85) -> (10.02, -12.85)
  line L198 (10.02, -18.85) -> (9.32, -18.85)
  line L199 (8.32, -18.85) -> (4.72, -18.85)
  line L200 (3.72, -18.85) -> (3.02, -18.85)
  line L201 (6, 9.95) -> (6, 9.25)
  line L202 (6, 8.25) -> (6, 5.65)
  line L203 (6, 4.65) -> (6, 3.95)
  line L204 (0, 3.95) -> (0, 6.45)
  line L205 (0, 7.45) -> (0, 9.95)
  line L206 (6, 30.65) -> (6, 29.95)
  line L207 (6, 35.95) -> (6, 35.25)
  line L208 (6, 34.25) -> (6, 31.65)
  line L209 (0, 29.95) -> (0, 32.45)
  line L210 (0, 33.45) -> (0, 35.95)
  line L211 (57.8, 29.95) -> (51.8, 29.95)
  line L212 (51.8, 9.95) -> (57.8, 9.95)
  line L213 (57.8, 29.25) -> (57.6, 29.25)
  line L214 (57.6, 29.25) -> (57.6, 28.25)
  line L215 (57.6, 28.25) -> (57.8, 28.25)
  line L216 (57.8, 11.65) -> (57.6, 11.65)
  line L217 (57.6, 11.65) -> (57.6, 10.65)
  line L218 (57.6, 10.65) -> (57.8, 10.65)
  line L219 (51.8, 20.05) -> (52, 20.05)
  line L220 (52, 20.05) -> (52, 19.05)
  line L221 (52, 19.05) -> (51.8, 19.05)
  line L222 (57.8, 29.25) -> (57.8, 29.95)
  line L223 (57.8, 9.95) -> (57.8, 10.65)
  line L224 (57.8, 11.65) -> (57.8, 28.25)
  line L225 (51.8, 29.95) -> (51.8, 20.05)
  line L226 (51.8, 19.05) -> (51.8, 9.95)
  line L227 (57.8, 29.95) -> (57.8, 15.0823) construction
  line L228 (57.8, 15.0823) -> (57.8, 9.95) construction
  point P0 (57.8, 19.95)
  dimension "d49" = 81.6
  dimension "d50" = 6
  dimension "d51" = 2
  dimension "d52" = 12.82
  dimension "d53" = 7
  dimension "d54" = 7
  dimension "d55" = 7
  dimension "d56" = 7
  dimension "d57" = 45.46
  dimension "d58" = 29.14
  dimension "d59" = 61.78
  dimension "d140" = 1
  dimension "d141" = 1
  dimension "d142" = 1
  dimension "d143" = 0.2
  dimension "d144" = 0.2
  dimension "d145" = 0.7
  dimension "d146" = 0.7
  dimension "d147" = 2.5
  dimension "d148" = 6
  dimension "d149" = 0.7
  dimension "d150" = 0.7
  dimension "d151" = 1
  dimension "d152" = 1
  dimension "d153" = 1
  dimension "d154" = 0.2
  dimension "d155" = 0.2
  dimension "d156" = 2.5
  dimension "d157" = 1
  dimension "d158" = 1
  dimension "d159" = 1
  dimension "d160" = 0.2
  dimension "d161" = 0.2
  dimension "d162" = 0.7
  dimension "d163" = 0.7
  dimension "d164" = 3
  dimension "d165" = 0.7
  dimension "d166" = 0.7
  dimension "d167" = 3
  dimension "d168" = 0.7
  dimension "d169" = 0.7
  dimension "d170" = 3
  dimension "d171" = 0.7
  dimension "d172" = 0.7
  dimension "d173" = 3
  dimension "d272" = 20
  dimension "d273" = 6
  dimension "d274" = 0.2
  dimension "d275" = 0.2
  dimension "d276" = 1
  dimension "d277" = 0.7
  dimension "d278" = 0.7
  dimension "d279" = 9.9
  dimension "d280" = 20
  constraints: 402 end point, 130 perpendicular, 64 symmetric about line, 39 parallel, 36 point on line, 34 collinear, 16 equal length, 15 horizontal, 7 vertical, 1 coincident, 1 midpoint
  measures "d49" distance of L2.start L6.end
  measures "d50" distance of L38.start L38.end
  measures "d51" vertical distance of L6.end L38.end
  measures "d52" horizontal distance of L43.start L2.start
  measures "d53" distance of L44.end L43.start
  measures "d54" distance of L42.end L41.start
  measures "d55" distance of L40.end L39.start
  measures "d56" distance of L38.end L37.start
  measures "d57" distance between parallel lines of L2 L39
  measures "d58" distance between parallel lines of L2 L41
  measures "d59" distance between parallel lines of L2 L37
  measures "d140" distance of L60.end L61.end
  measures "d141" distance of L63.end L64.end
  measures "d142" distance of L66.end L67.end
  measures "d143" distance of L67.end L68.end
  measures "d144" distance of L61.end L62.end
  measures "d145" vertical distance of L52.end L60.end
  measures "d146" vertical distance of L49.end L64.end
  measures "d147" vertical distance of L51.start L66.end
  measures "d148" distance of L51.start L49.start
  measures "d149" vertical distance of L56.end L71.end
  measures "d150" vertical distance of L55.start L75.end
  measures "d151" distance of L71.end L72.end
  measures "d152" distance of L74.end L75.end
  measures "d153" distance of L77.end L78.end
  measures "d154" distance of L72.end L73.end
  measures "d155" distance of L78.end L79.end
  measures "d156" vertical distance of L56.start L77.end
  measures "d157" distance of L81.end L82.end
  measures "d158" distance of L87.end L88.end
  measures "d159" distance of L84.end L85.end
  measures "d160" distance of L85.end L86.end
  measures "d161" distance of L88.end L89.end
  measures "d162" horizontal distance of L38.end L81.end
  measures "d163" horizontal distance of L37.start L85.end
  measures "d164" horizontal distance of L38.start L87.end
  measures "d165" horizontal distance of L44.end L108.end
  measures "d166" horizontal distance of L43.start L112.end
  measures "d167" horizontal distance of L43.end L115.end
  measures "d168" horizontal distance of L41.start L103.end
  measures "d169" horizontal distance of L42.end L99.end
  measures "d170" horizontal distance of L41.end L105.end
  measures "d171" horizontal distance of L39.start L94.end
  measures "d172" horizontal distance of L40.end L90.end
  measures "d173" horizontal distance of L40.start L96.end
  measures "d272" distance of L212.end L211.start
  measures "d273" distance of L212.start L212.end
  measures "d274" distance of L214.end L215.end
  measures "d275" distance of L220.end L221.end
  measures "d276" distance of L213.end L214.end
  measures "d277" vertical distance of L211.start L213.end
  measures "d278" vertical distance of L212.end L217.end
  measures "d279" vertical distance of L211.end L219.end
  measures "d280" distance from line of L45 L211.end
extrude "Extrusion6" add sketch "Esquisse8" against normal blind 6 separate body
ref_plane "Plan de construction3" through (32, -1, -9.8) normal (1, 0, 0) x (0, 0, -1)
mirror "Symétrie3" about plane through (32, -1, -9.8) normal (1, 0, 0) of "Extrusion6" bodies 3
sketch "Esquisse9" plane through (28.5, -26.9, 6) normal (0, -1, 0) x (1, 0, 0)
  line L0 (27.4, -6) -> (20.4, -6) construction
  line L1 (27.4, -6) -> (27.4, -0.5)
  line L2 (20.4, 0) -> (27.4, 0) projected
  line L3 (26.9, 0) -> (20.9, 0)
  line L4 (20.4, 0) -> (20.4, -6) projected
  line L5 (20.4, -0.5) -> (20.4, -6)
  line L6 (-13.4, -6) -> (-20.4, -6) construction
  line L7 (-20.4, 0) -> (-13.4, 0) projected
  line L8 (-13.4, -6) -> (-13.4, -0.5)
  line L9 (-20.4, 0) -> (-20.4, -6) projected
  line L10 (-13.9, 0) -> (-19.9, 0)
  line L11 (-20.4, -0.5) -> (-20.4, -6)
  line L12 (-20.4, -6) -> (-31.3, -6)
  line L13 (38.3, -6) -> (27.4, -6)
  line L14 (6.5, -16) -> (3.5, -16)
  line L15 (3.5, -16) -> (0.5, -16)
  line L16 (-11.5, -6) -> (18.5, -6) construction
  line L17 (3.5, 17.52) -> (3.5, -105.12) projected
  line L18 (20.4, -6) -> (6.5, -6)
  line L19 (0.5, -6) -> (-13.4, -6)
  line L20 (-13.4, -0.5) -> (-13.9, 0)
  line L21 (-19.9, 0) -> (-20.4, -0.5)
  line L22 (20.9, 0) -> (20.4, -0.5)
  line L23 (27.4, -0.5) -> (26.9, 0)
  line L24 (6.5, -6.7) -> (6.3, -6.7)
  line L25 (6.3, -6.7) -> (6.3, -7.7)
  line L26 (6.3, -7.7) -> (6.5, -7.7)
  line L27 (6.5, -15.3) -> (6.3, -15.3)
  line L28 (6.3, -15.3) -> (6.3, -14.3)
  line L29 (0.5, -10.5) -> (0.7, -10.5)
  line L30 (0.7, -10.5) -> (0.7, -11.5)
  line L31 (0.7, -11.5) -> (0.5, -11.5)
  line L32 (6.3, -14.3) -> (6.5, -14.3)
  line L33 (6.5, -15.3) -> (6.5, -16)
  line L34 (6.5, -6) -> (6.5, -6.7)
  line L35 (6.5, -7.7) -> (6.5, -14.3)
  line L36 (0.5, -16) -> (0.5, -11.5)
  line L37 (0.5, -10.5) -> (0.5, -6)
  line L38 (38.3, -6) -> (38.3, -18.82)
  line L39 (38.3, -18.82) -> (43.8, -18.82)
  line L40 (44.3, -22.82) -> (44.3, -25.82) projected
  line L41 (44.3, -19.32) -> (44.3, -25.32)
  line L42 (38.3, -25.82) -> (38.3, -22.82) projected
  line L43 (43.8, -25.82) -> (38.3, -25.82)
  line L44 (38.3, -38.14) -> (38.3, -35.14) projected
  line L45 (38.3, -25.82) -> (38.3, -35.14)
  line L46 (44.3, -35.14) -> (38.3, -35.14) projected
  line L47 (38.3, -35.14) -> (43.8, -35.14)
  line L48 (44.3, -39.14) -> (44.3, -42.14) projected
  line L49 (44.3, -35.64) -> (44.3, -41.64)
  line L50 (38.3, -42.14) -> (38.3, -39.14) projected
  line L51 (43.8, -42.14) -> (38.3, -42.14)
  line L52 (44.3, -51.46) -> (38.3, -51.46) projected
  line L53 (38.3, -42.14) -> (38.3, -51.46)
  line L54 (44.3, -51.46) -> (44.3, -54.46) projected
  line L55 (38.3, -51.46) -> (43.8, -51.46)
  line L56 (44.3, -51.96) -> (44.3, -57.96)
  line L57 (44.3, -58.46) -> (38.3, -58.46) projected
  line L58 (43.8, -58.46) -> (38.3, -58.46)
  line L59 (38.3, -70.78) -> (38.3, -67.78) projected
  line L60 (38.3, -58.46) -> (38.3, -67.78)
  line L61 (44.3, -67.78) -> (44.3, -70.78) projected
  line L62 (38.3, -67.78) -> (43.8, -67.78)
  line L63 (44.3, -74.78) -> (38.3, -74.78) projected
  line L64 (44.3, -68.28) -> (44.3, -74.28)
  line L65 (43.8, -74.78) -> (38.3, -74.78)
  line L66 (38.3, -74.78) -> (38.3, -87.6)
  line L67 (38.3, -87.6) -> (-31.3, -87.6)
  line L68 (-31.3, -87.6) -> (-31.3, -74.78)
  line L69 (-37.3, -71.78) -> (-37.3, -74.78) projected
  line L70 (-31.3, -74.78) -> (-36.8, -74.78)
  line L71 (-37.3, -67.78) -> (-31.3, -67.78) projected
  line L72 (-37.3, -74.28) -> (-37.3, -68.28)
  line L73 (-36.8, -67.78) -> (-31.3, -67.78)
  line L74 (-37.3, -58.46) -> (-31.3, -58.46) projected
  line L75 (-31.3, -67.78) -> (-31.3, -58.46)
  line L76 (-31.3, -58.46) -> (-36.8, -58.46)
  line L77 (-37.3, -57.96) -> (-37.3, -51.96)
  line L78 (-36.8, -51.46) -> (-31.3, -51.46)
  line L79 (-31.3, -42.14) -> (-31.3, -39.14) projected
  line L80 (-31.3, -51.46) -> (-31.3, -42.14)
  line L81 (-37.3, -42.14) -> (-31.3, -42.14) projected
  line L82 (-31.3, -42.14) -> (-36.8, -42.14)
  line L83 (-37.3, -41.64) -> (-37.3, -35.64)
  line L84 (-31.3, -38.14) -> (-31.3, -35.14) projected
  line L85 (-36.8, -35.14) -> (-31.3, -35.14)
  line L86 (-31.3, -35.14) -> (-31.3, -25.82)
  line L87 (-37.3, -25.82) -> (-31.3, -25.82) projected
  line L88 (-31.3, -25.82) -> (-36.8, -25.82)
  line L89 (-37.3, -25.32) -> (-37.3, -19.32)
  line L90 (-37.3, -18.82) -> (-31.3, -18.82) projected
  line L91 (-36.8, -18.82) -> (-31.3, -18.82)
  line L92 (-31.3, -18.82) -> (-31.3, -6)
  line L93 (44.3, -74.28) -> (43.8, -74.78)
  line L94 (44.3, -68.28) -> (43.8, -67.78)
  line L95 (44.3, -57.96) -> (43.8, -58.46)
  line L96 (44.3, -51.96) -> (43.8, -51.46)
  line L97 (44.3, -41.64) -> (43.8, -42.14)
  line L98 (43.8, -35.14) -> (44.3, -35.64)
  line L99 (44.3, -25.32) -> (43.8, -25.82)
  line L100 (43.8, -18.82) -> (44.3, -19.32)
  line L101 (-37.3, -25.32) -> (-36.8, -25.82)
  line L102 (-37.3, -19.32) -> (-36.8, -18.82)
  line L103 (-37.3, -35.64) -> (-36.8, -35.14)
  line L104 (-37.3, -41.64) -> (-36.8, -42.14)
  line L105 (-36.8, -51.46) -> (-37.3, -51.96)
  line L106 (-37.3, -57.96) -> (-36.8, -58.46)
  line L107 (-37.3, -74.28) -> (-36.8, -74.78)
  line L108 (-36.8, -67.78) -> (-37.3, -68.28)
  point P0 (-28.5, -6)
  point P1 (44.3, -18.82)
  point P2 (-37.3, -51.46)
  point P3 (-37.3, -35.14)
  dimension "d80" = 6
  dimension "d81" = 10
  dimension "d206" = 0.5
  dimension "d207" = 0.5
  dimension "d208" = 0.5
  dimension "d209" = 0.5
  dimension "d210" = 0.5
  dimension "d211" = 0.5
  dimension "d212" = 0.5
  dimension "d213" = 0.5
  dimension "d214" = 1
  dimension "d215" = 1
  dimension "d216" = 1
  dimension "d217" = 0.2
  dimension "d218" = 0.2
  dimension "d219" = 0.7
  dimension "d220" = 0.7
  dimension "d221" = 4.5
  dimension "d222" = 0.5
  dimension "d223" = 0.5
  dimension "d224" = 0.5
  dimension "d225" = 0.5
  dimension "d226" = 0.5
  dimension "d227" = 0.5
  dimension "d228" = 0.5
  dimension "d229" = 0.5
  dimension "d230" = 0.5
  dimension "d231" = 0.5
  dimension "d232" = 0.5
  dimension "d233" = 0.5
  dimension "d234" = 0.5
  dimension "d235" = 0.5
  dimension "d236" = 0.5
  dimension "d237" = 0.5
  dimension "d238" = 0.5
  dimension "d239" = 0.5
  dimension "d240" = 0.5
  dimension "d241" = 0.5
  dimension "d242" = 0.5
  dimension "d243" = 0.5
  dimension "d244" = 0.5
  dimension "d245" = 0.5
  dimension "d246" = 0.5
  dimension "d247" = 0.5
  dimension "d248" = 0.5
  dimension "d249" = 0.5
  dimension "d250" = 0.5
  dimension "d251" = 0.5
  dimension "d252" = 0.5
  dimension "d253" = 0.5
  constraints: 162 end point, 56 perpendicular, 45 point on line, 13 collinear, 4 horizontal, 2 vertical
  measures "d80" distance of L15.end L14.start
  measures "d81" distance of L19.start L15.end
  measures "d206" distance of L8.end L7.end
  measures "d207" distance of L10.start L7.end
  measures "d208" distance of L10.end L7.start
  measures "d209" distance of L11.start L7.start
  measures "d210" distance of L3.end L2.start
  measures "d211" distance of L5.start L2.start
  measures "d212" distance of L1.end L2.end
  measures "d213" distance of L3.start L2.end
  measures "d214" distance of L27.end L28.end
  measures "d215" distance of L29.end L30.end
  measures "d216" distance of L24.end L25.end
  measures "d217" distance of L25.end L26.end
  measures "d218" distance of L29.start L29.end
  measures "d219" vertical distance of L14.start L27.end
  measures "d220" vertical distance of L18.end L24.end
  measures "d221" vertical distance of L19.start L29.end
  measures "d222" distance of L64.end L63.start
  measures "d223" distance of L65.start L63.start
  measures "d224" distance of L64.start L61.start
  measures "d225" distance of L62.end L61.start
  measures "d226" distance of L56.end L57.start
  measures "d227" distance of L58.start L57.start
  measures "d228" distance of L56.start L52.start
  measures "d229" distance of L55.end L52.start
  measures "d230" distance of L49.end L48.end
  measures "d231" distance of L51.start L48.end
  measures "d232" distance of L47.end L46.start
  measures "d233" distance of L49.start L46.start
  measures "d234" distance of L41.end L40.end
  measures "d235" distance of L43.start L40.end
  measures "d236" distance of L39.end point (44.3, -18.82)
  measures "d237" distance of L41.start point (44.3, -18.82)
  measures "d238" distance of L89.start L87.start
  measures "d239" distance of L88.end L87.start
  measures "d240" distance of L89.end L90.start
  measures "d241" distance of L91.start L90.start
  measures "d242" distance of L83.end point (-37.3, -35.14)
  measures "d243" distance of L85.start point (-37.3, -35.14)
  measures "d244" distance of L83.start L81.start
  measures "d245" distance of L82.end L81.start
  measures "d246" distance of L78.start point (-37.3, -51.46)
  measures "d247" distance of L77.end point (-37.3, -51.46)
  measures "d248" distance of L77.start L74.start
  measures "d249" distance of L76.end L74.start
  measures "d250" distance of L72.start L69.end
  measures "d251" distance of L70.end L69.end
  measures "d252" distance of L73.start L71.start
  measures "d253" distance of L72.end L71.start
extrude "Extrusion7" add sketch "Esquisse9" along normal blind 6 separate body contours L13 L38 L39 L100 L41 L40 L99 L43 L45 L46 L98 L49 L48 L97 L51 L53 L52 L96 L54 L56 L95 L57 L60 L62 L94 L61 L64 L93 L63 L66 L67 L17 L14 L33 L27 L28 L32 L35 L26 L25 L24 L34 L18 L4 L22 L2 L23 L1 | L17 L67 L68 L70 L107 L69 L72 L108 L71 L75 L74 L106 L77 L105 L78 L80 L81 L104 L83 L103 L85 L86 L87 L101 L89 L102 L90 L92 L12 L9 L21 L7 L20 L8 L19 L37 L29 L30 L31 L36 L15
ref_plane "Plan de construction4" through (-10.8, 5.9, -9.8) normal (0, 1, 0) x (1, 0, 0)
mirror "Symétrie4" about plane through (-10.8, 5.9, -9.8) normal (0, 1, 0) of "Extrusion7" bodies 4
sketch "Esquisse10" plane through (72.8, -34.9, -81.6) normal (0, 0, -1) x (-1, 0, 0)
  line L0 (81.6, 81.6) -> (0, 81.6) projected
  line L1 (81.6, 0) -> (0, 0) projected
  line L2 (0, 81.6) -> (81.6, 81.6)
  line L3 (81.6, 81.6) -> (81.6, 0)
  line L4 (81.6, 0) -> (0, 0)
  line L5 (0, 0) -> (0, 81.6)
  point P0 (72.8, 34.9)
  constraints: 8 end point, 2 parallel, 1 horizontal, 1 perpendicular
extrude "Extrusion8" add sketch "Esquisse10" along normal blind 6 separate body
sketch "Esquisse12" plane through (72.8, -34.9, -81.6) normal (0, 0, 1) x (1, 0, 0)
  line L0 (-75.6, 8) -> (-75.6, 2) projected
  line L1 (-75.6, 8) -> (-6, 8)
  line L2 (-6, 8) -> (-6, 73.6)
  line L3 (-6, 73.6) -> (-75.6, 73.6)
  line L4 (-75.6, 73.6) -> (-75.6, 8)
  point P0 (-72.8, 34.9)
  constraints: 8 end point, 2 parallel, 1 horizontal, 1 perpendicular
extrude "Extrusion10" add sketch "Esquisse12" along normal blind 6 separate body